Cycloid_R27_Rr3_N12_E1.3 v13 (Autodesk Fusion 360 design; units mm, degrees)
Autodesk Fusion 360 part; units mm, degrees
sketch "Cycloid_R27_Rr3_N12_E1.3" plane through (0, 0, 0) normal (0, 0, 1) x (1, 0, 0)
  spline S0 degree 3 poles (22.7, 0) (22.7, 0.6125) (22.8641, 1.1792) (23.0258, 1.5653) (23.2959, 2.21) (23.5195, 2.5021) (23.6979, 2.8113) (23.9582, 3.2623) (24.184, 3.7168) (24.3374, 4.3219) (24.5549, 5.1798) (24.5562, 6.3107) (24.2085, 7.3389) (23.915, 8.2071) (23.3942, 8.9658) (22.849, 9.4857) (22.4062, 9.9079) (21.976, 10.1744) (21.5331, 10.4069) (21.2661, 10.5471) (20.9901, 10.6664) (20.5771, 10.9051) (20.2716, 11.0818) (19.8561, 11.3456) (19.4485, 11.8071) (19.0699, 12.2358) (18.7698, 12.8235) (18.6313, 13.3021) (18.4366, 13.9744) (18.4464, 14.4072) (18.4331, 14.7458) (18.4124, 15.2731) (18.4019, 15.6633) (18.3082, 16.1442) (18.1696, 16.8555) (17.8268, 17.7143) (17.2032, 18.47) (16.54, 19.2736) (15.5782, 19.8983) (14.6774, 20.1844) (14.0278, 20.3907) (13.4343, 20.4394) (12.9166, 20.4231) (12.5338, 20.411) (12.2077, 20.3607) (11.6984, 20.3178) (11.348, 20.2882) (10.8614, 20.2427) (10.1869, 20.3943) (9.6219, 20.5214) (8.984, 20.8456) (8.564, 21.1934) (8.0345, 21.632) (7.7911, 22.0076) (7.5955, 22.2842) (7.2871, 22.7202) (7.0844, 23.0287) (6.7768, 23.3686) (6.3145, 23.8797) (5.6298, 24.415) (4.747, 24.748) (3.7861, 25.1104) (2.6334, 25.1828) (1.6851, 24.9763) (1.0227, 24.8321) (0.4702, 24.5758) (0.0307, 24.2999) (-0.3331, 24.0715) (-0.6042, 23.843) (-0.9968, 23.5316) (-1.2336, 23.3438) (-1.5241, 23.0997) (-2.0364, 22.845) (-2.4624, 22.6331) (-3.0792, 22.4489) (-3.6623, 22.4317) (-4.2859, 22.4133) (-4.7902, 22.5464) (-5.1412, 22.6614) (-5.7453, 22.8593) (-6.0464, 23.0205) (-6.4003, 23.1512) (-6.9273, 23.3459) (-7.5288, 23.5011) (-8.2685, 23.5031) (-9.1925, 23.5056) (-10.2849, 23.2163) (-11.164, 22.6594) (-11.975, 22.1456) (-12.5739, 21.4439) (-12.9316, 20.8087) (-13.1579, 20.4068) (-13.2952, 20.0445) (-13.4326, 19.6384) (-13.5351, 19.3355) (-13.6176, 18.9984) (-13.88, 18.4589) (-14.0614, 18.0859) (-14.3743, 17.5893) (-14.8368, 17.1805) (-15.3004, 16.7706) (-15.8457, 16.5145) (-16.2496, 16.3807) (-16.9256, 16.1568) (-17.2959, 16.1359) (-17.6504, 16.0674) (-18.1624, 15.9683) (-18.6562, 15.8398) (-19.2159, 15.5567) (-19.9761, 15.1721) (-20.7954, 14.4746) (-21.3419, 13.5856) (-21.8985, 12.6803) (-22.1404, 11.6323) (-22.1375, 10.7953) (-22.1357, 10.2824) (-22.0608, 9.8568) (-21.9594, 9.4298) (-21.8808, 9.099) (-21.7667, 8.7789) (-21.6764, 8.1745) (-21.6194, 7.793) (-21.5831, 7.2498) (-21.7151, 6.6502) (-21.8449, 6.0605) (-22.143, 5.5032) (-22.4147, 5.1385) (-22.8549, 4.5478) (-23.1744, 4.3137) (-23.4331, 4.0707) (-23.8211, 3.7064) (-24.1569, 3.3625) (-24.4808, 2.8538) (-24.9221, 2.1607) (-25.272, 1.1745) (-25.2982, 0.1386) (-25.3223, -0.8106) (-25.0739, -1.7578) (-24.7014, -2.4719) (-24.3965, -3.0566) (-24.0398, -3.477) (-23.6716, -3.8416) (-23.4461, -4.065) (-23.2125, -4.2595) (-22.876, -4.6039) (-22.6373, -4.8482) (-22.3173, -5.1939) (-22.0405, -5.74) (-21.7861, -6.2422) (-21.6353, -6.8982) (-21.625, -7.4159) (-21.6112, -8.1077) (-21.7373, -8.5368) (-21.8186, -8.8665) (-21.9475, -9.3885) (-22.0486, -9.7489) (-22.1025, -10.2133) (-22.1829, -10.9066) (-22.1299, -11.7884) (-21.7892, -12.6793) (-21.4199, -13.6452) (-20.7045, -14.5555) (-19.9227, -15.1243) (-19.3974, -15.5065) (-18.8642, -15.7434) (-18.3853, -15.8897) (-17.9769, -16.0144) (-17.6277, -16.07) (-17.1406, -16.1615) (-16.8439, -16.2172) (-16.4707, -16.276) (-15.9426, -16.4947) (-15.5053, -16.6757) (-14.9625, -17.0173) (-14.5654, -17.4455) (-14.1421, -17.9021) (-13.9093, -18.3711) (-13.765, -18.7126) (-13.5164, -19.301) (-13.4413, -19.6348) (-13.3093, -19.987) (-13.1131, -20.5104) (-12.8409, -21.0621) (-12.3647, -21.6203) (-11.7686, -22.3192) (-10.8433, -22.9587) (-9.8503, -23.2649) (-8.9138, -23.5536) (-7.9704, -23.5471) (-7.2443, -23.3971) (-6.7961, -23.3044) (-6.4349, -23.1714) (-6.0396, -23.0098) (-5.7254, -22.8814) (-5.397, -22.7049) (-4.742, -22.5476) (-4.3177, -22.4458) (-3.7077, -22.3819) (-3.1052, -22.4891) (-2.4937, -22.5979) (-1.9804, -22.8541) (-1.6382, -23.069) (-1.0631, -23.4303) (-0.813, -23.6841) (-0.5276, -23.9055) (-0.0967, -24.2396) (0.3681, -24.5462) (1.0085, -24.7802) (1.8665, -25.0938) (3.0127, -25.2008) (4.0658, -24.9549) (4.945, -24.7496) (5.7243, -24.3197) (6.2774, -23.8522) (6.7357, -23.4649) (7.0339, -23.0841) (7.3327, -22.66) (7.5073, -22.4123) (7.6728, -22.1364) (8.0197, -21.732) (8.2737, -21.436) (8.6677, -21.048) (9.2148, -20.7552) (9.7556, -20.4658) (10.3782, -20.3321) (10.8314, -20.3024) (11.5372, -20.2561) (11.9151, -20.3387) (12.2602, -20.3744) (12.7705, -20.4273) (13.2294, -20.4562) (13.7969, -20.3811) (14.601, -20.2747) (15.574, -19.9156) (16.3855, -19.2718) (17.1618, -18.6559) (17.7486, -17.8083) (18.0529, -17.027) (18.2904, -16.4172) (18.3721, -15.8769) (18.4057, -15.3617) (18.4274, -15.0299) (18.417, -14.7129) (18.468, -14.1849) (18.5019, -13.8331) (18.5698, -13.3444) (18.8214, -12.7816) (19.0638, -12.2391) (19.4972, -11.7071) (19.886, -11.3825) (20.4355, -10.9236) (20.8302, -10.7624) (21.1363, -10.6086) (21.5943, -10.3785) (21.9506, -10.1986) (22.3517, -9.903) (22.9505, -9.4617) (23.5934, -8.7583) (24.0064, -7.8502) (24.438, -6.9014) (24.5746, -5.7752) (24.443, -4.8563) (24.3415, -4.1467) (24.1137, -3.5815) (23.8589, -3.1009) (23.7019, -2.8048) (23.5323, -2.548) (23.3033, -2.1326) (23.1455, -1.8464) (22.9357, -1.4585) (22.8, -0.8709) (22.7389, -0.6059) (22.7, -0.3041) (22.7, 0) knots 0 0 0 0 0.03430611 0.03430611 0.03430611 0.09160089 0.09160089 0.09160089 0.17516843 0.17516843 0.17516843 0.29364805 0.29364805 0.29364805 0.39367837 0.39367837 0.39367837 0.47491142 0.47491142 0.47491142 0.5238857 0.5238857 0.5238857 0.5601117 0.5601117 0.5601117 0.59375346 0.59375346 0.59375346 0.64102096 0.64102096 0.64102096 0.71462274 0.71462274 0.71462274 0.82350645 0.82350645 0.82350645 0.93929104 0.93929104 0.93929104 1.02278938 1.02278938 1.02278938 1.08452204 1.08452204 1.08452204 1.12698868 1.12698868 1.12698868 1.16256928 1.16256928 1.16256928 1.2074329 1.2074329 1.2074329 1.27813427 1.27813427 1.27813427 1.38442402 1.38442402 1.38442402 1.50011681 1.50011681 1.50011681 1.58093887 1.58093887 1.58093887 1.64783508 1.64783508 1.64783508 1.68819847 1.68819847 1.68819847 1.72176401 1.72176401 1.72176401 1.75766421 1.75766421 1.75766421 1.81944996 1.81944996 1.81944996 1.91144577 1.91144577 1.91144577 2.02636364 2.02636364 2.02636364 2.13238209 2.13238209 2.13238209 2.19946819 2.19946819 2.19946819 2.24950351 2.24950351 2.24950351 2.28408659 2.28408659 2.28408659 2.31875688 2.31875688 2.31875688 2.37677319 2.37677319 2.37677319 2.46056379 2.46056379 2.46056379 2.57436902 2.57436902 2.57436902 2.69026953 2.69026953 2.69026953 2.7613022 2.7613022 2.7613022 2.81633163 2.81633163 2.81633163 2.85106272 2.85106272 2.85106272 2.88522235 2.88522235 2.88522235 2.94055461 2.94055461 2.94055461 3.02352207 3.02352207 3.02352207 3.13655488 3.13655488 3.13655488 3.24012125 3.24012125 3.24012125 3.32490764 3.32490764 3.32490764 3.37684352 3.37684352 3.37684352 3.413689 3.413689 3.413689 3.44756834 3.44756834 3.44756834 3.49284999 3.49284999 3.49284999 3.56456328 3.56456328 3.56456328 3.67163442 3.67163442 3.67163442 3.78772273 3.78772273 3.78772273 3.86570593 3.86570593 3.86570593 3.93220732 3.93220732 3.93220732 3.97271018 3.97271018 3.97271018 4.00624962 4.00624962 4.00624962 4.04200453 4.04200453 4.04200453 4.10360991 4.10360991 4.10360991 4.19515686 4.19515686 4.19515686 4.30976018 4.30976018 4.30976018 4.41784404 4.41784404 4.41784404 4.48458241 4.48458241 4.48458241 4.53760721 4.53760721 4.53760721 4.57196123 4.57196123 4.57196123 4.60683368 4.60683368 4.60683368 4.66544576 4.66544576 4.66544576 4.75391117 4.75391117 4.75391117 4.87242781 4.87242781 4.87242781 4.9713785 4.9713785 4.9713785 5.05336643 5.05336643 5.05336643 5.10124548 5.10124548 5.10124548 5.1362929 5.1362929 5.1362929 5.17093432 5.17093432 5.17093432 5.22489121 5.22489121 5.22489121 5.30468399 5.30468399 5.30468399 5.41776894 5.41776894 5.41776894 5.52594598 5.52594598 5.52594598 5.61037845 5.61037845 5.61037845 5.66476024 5.66476024 5.66476024 5.70099726 5.70099726 5.70099726 5.7359224 5.7359224 5.7359224 5.78528307 5.78528307 5.78528307 5.85915785 5.85915785 5.85915785 5.96942398 5.96942398 5.96942398 6.08463245 6.08463245 6.08463245 6.17359078 6.17359078 6.17359078 6.22838805 6.22838805 6.22838805 6.26615392 6.26615392 6.26615392 6.28318531 6.28318531 6.28318531 6.28318531
  circle A0 centre (0, 0) radius 9.1
  circle A1 centre (0, 0) radius 16 construction
  line L0 (0, 0) -> (0, 22.3554) construction
  circle A2 centre (0, 16) radius 4.3
  circle A3 centre (-15.2169, 4.9443) radius 4.3
  circle A4 centre (-9.4046, -12.9443) radius 4.3
  circle A5 centre (9.4046, -12.9443) radius 4.3
  circle A6 centre (15.2169, 4.9443) radius 4.3
  circle A7 centre (0, 0) radius 8
  dimension "d13" = 18.2
  dimension "d14" = 8.6
  dimension "d16" = 360
  dimension "d17" = 16
  dimension "d28" = 32
  constraint coincident A0.centre A1.centre
  constraint vertical L0
  constraint coincident A1 A2.centre
  constraint coincident L0 A2.centre
  constraint concentric A0 A7
  measures "d13" diameter of A0
  measures "d14" diameter of A2
  measures "d17" diameter of A7
  measures "d28" diameter of A1
extrude "Extrude3" add sketch "Cycloid_R27_Rr3_N12_E1.3" along normal blind 8 contours S0 makes body 1
extrude "Extrude4" add sketch "Cycloid_R27_Rr3_N12_E1.3" along normal blind 1.8 contours A0 bodies 1
sketch "Sketch4" plane through (0, 0, 8) normal (0, 0, 1) x (-1, 0, 0)
  circle A0 centre (0, 0) radius 9.1
  circle A1 centre (9.4046, 12.9443) radius 4.3
  circle A2 centre (15.2169, -4.9443) radius 4.3
  circle A3 centre (0, -16) radius 4.3
  circle A4 centre (-9.4046, 12.9443) radius 4.3
  circle A5 centre (-15.2169, -4.9443) radius 4.3
  spline S0 degree 3 poles (-22.7, 0) (-22.7, -0.6125) (-22.8641, -1.1792) (-23.0258, -1.5653) (-23.2959, -2.21) (-23.5195, -2.5021) (-23.6979, -2.8113) (-23.9582, -3.2623) (-24.184, -3.7168) (-24.3374, -4.3219) (-24.5549, -5.1798) (-24.5562, -6.3107) (-24.2085, -7.3389) (-23.915, -8.2071) (-23.3942, -8.9658) (-22.849, -9.4857) (-22.4062, -9.9079) (-21.976, -10.1744) (-21.5331, -10.4069) (-21.2661, -10.5471) (-20.9901, -10.6664) (-20.5771, -10.9051) (-20.2716, -11.0818) (-19.8561, -11.3456) (-19.4485, -11.8071) (-19.0699, -12.2358) (-18.7698, -12.8235) (-18.6313, -13.3021) (-18.4366, -13.9744) (-18.4464, -14.4072) (-18.4331, -14.7458) (-18.4124, -15.2731) (-18.4019, -15.6633) (-18.3082, -16.1442) (-18.1696, -16.8555) (-17.8268, -17.7143) (-17.2032, -18.47) (-16.54, -19.2736) (-15.5782, -19.8983) (-14.6774, -20.1844) (-14.0278, -20.3907) (-13.4343, -20.4394) (-12.9166, -20.4231) (-12.5338, -20.411) (-12.2077, -20.3607) (-11.6984, -20.3178) (-11.348, -20.2882) (-10.8614, -20.2427) (-10.1869, -20.3943) (-9.6219, -20.5214) (-8.984, -20.8456) (-8.564, -21.1934) (-8.0345, -21.632) (-7.7911, -22.0076) (-7.5955, -22.2842) (-7.2871, -22.7202) (-7.0844, -23.0287) (-6.7768, -23.3686) (-6.3145, -23.8797) (-5.6298, -24.415) (-4.747, -24.748) (-3.7861, -25.1104) (-2.6334, -25.1828) (-1.6851, -24.9763) (-1.0227, -24.8321) (-0.4702, -24.5758) (-0.0307, -24.2999) (0.3331, -24.0715) (0.6042, -23.843) (0.9968, -23.5316) (1.2336, -23.3438) (1.5241, -23.0997) (2.0364, -22.845) (2.4624, -22.6331) (3.0792, -22.4489) (3.6623, -22.4317) (4.2859, -22.4133) (4.7902, -22.5464) (5.1412, -22.6614) (5.7453, -22.8593) (6.0464, -23.0205) (6.4003, -23.1512) (6.9273, -23.3459) (7.5288, -23.5011) (8.2685, -23.5031) (9.1925, -23.5056) (10.2849, -23.2163) (11.164, -22.6594) (11.975, -22.1456) (12.5739, -21.4439) (12.9316, -20.8087) (13.1579, -20.4068) (13.2952, -20.0445) (13.4326, -19.6384) (13.5351, -19.3355) (13.6176, -18.9984) (13.88, -18.4589) (14.0614, -18.0859) (14.3743, -17.5893) (14.8368, -17.1805) (15.3004, -16.7706) (15.8457, -16.5145) (16.2496, -16.3807) (16.9256, -16.1568) (17.2959, -16.1359) (17.6504, -16.0674) (18.1624, -15.9683) (18.6562, -15.8398) (19.2159, -15.5567) (19.9761, -15.1721) (20.7954, -14.4746) (21.3419, -13.5856) (21.8985, -12.6803) (22.1404, -11.6323) (22.1375, -10.7953) (22.1357, -10.2824) (22.0608, -9.8568) (21.9594, -9.4298) (21.8808, -9.099) (21.7667, -8.7789) (21.6764, -8.1745) (21.6194, -7.793) (21.5831, -7.2498) (21.7151, -6.6502) (21.8449, -6.0605) (22.143, -5.5032) (22.4147, -5.1385) (22.8549, -4.5478) (23.1744, -4.3137) (23.4331, -4.0707) (23.8211, -3.7064) (24.1569, -3.3625) (24.4808, -2.8538) (24.9221, -2.1607) (25.272, -1.1745) (25.2982, -0.1386) (25.3223, 0.8106) (25.0739, 1.7578) (24.7014, 2.4719) (24.3965, 3.0566) (24.0398, 3.477) (23.6716, 3.8416) (23.4461, 4.065) (23.2125, 4.2595) (22.876, 4.6039) (22.6373, 4.8482) (22.3173, 5.1939) (22.0405, 5.74) (21.7861, 6.2422) (21.6353, 6.8982) (21.625, 7.4159) (21.6112, 8.1077) (21.7373, 8.5368) (21.8186, 8.8665) (21.9475, 9.3885) (22.0486, 9.7489) (22.1025, 10.2133) (22.1829, 10.9066) (22.1299, 11.7884) (21.7892, 12.6793) (21.4199, 13.6452) (20.7045, 14.5555) (19.9227, 15.1243) (19.3974, 15.5065) (18.8642, 15.7434) (18.3853, 15.8897) (17.9769, 16.0144) (17.6277, 16.07) (17.1406, 16.1615) (16.8439, 16.2172) (16.4707, 16.276) (15.9426, 16.4947) (15.5053, 16.6757) (14.9625, 17.0173) (14.5654, 17.4455) (14.1421, 17.9021) (13.9093, 18.3711) (13.765, 18.7126) (13.5164, 19.301) (13.4413, 19.6348) (13.3093, 19.987) (13.1131, 20.5104) (12.8409, 21.0621) (12.3647, 21.6203) (11.7686, 22.3192) (10.8433, 22.9587) (9.8503, 23.2649) (8.9138, 23.5536) (7.9704, 23.5471) (7.2443, 23.3971) (6.7961, 23.3044) (6.4349, 23.1714) (6.0396, 23.0098) (5.7254, 22.8814) (5.397, 22.7049) (4.742, 22.5476) (4.3177, 22.4458) (3.7077, 22.3819) (3.1052, 22.4891) (2.4937, 22.5979) (1.9804, 22.8541) (1.6382, 23.069) (1.0631, 23.4303) (0.813, 23.6841) (0.5276, 23.9055) (0.0967, 24.2396) (-0.3681, 24.5462) (-1.0085, 24.7802) (-1.8665, 25.0938) (-3.0127, 25.2008) (-4.0658, 24.9549) (-4.945, 24.7496) (-5.7243, 24.3197) (-6.2774, 23.8522) (-6.7357, 23.4649) (-7.0339, 23.0841) (-7.3327, 22.66) (-7.5073, 22.4123) (-7.6728, 22.1364) (-8.0197, 21.732) (-8.2737, 21.436) (-8.6677, 21.048) (-9.2148, 20.7552) (-9.7556, 20.4658) (-10.3782, 20.3321) (-10.8314, 20.3024) (-11.5372, 20.2561) (-11.9151, 20.3387) (-12.2602, 20.3744) (-12.7705, 20.4273) (-13.2294, 20.4562) (-13.7969, 20.3811) (-14.601, 20.2747) (-15.574, 19.9156) (-16.3855, 19.2718) (-17.1618, 18.6559) (-17.7486, 17.8083) (-18.0529, 17.027) (-18.2904, 16.4172) (-18.3721, 15.8769) (-18.4057, 15.3617) (-18.4274, 15.0299) (-18.417, 14.7129) (-18.468, 14.1849) (-18.5019, 13.8331) (-18.5698, 13.3444) (-18.8214, 12.7816) (-19.0638, 12.2391) (-19.4972, 11.7071) (-19.886, 11.3825) (-20.4355, 10.9236) (-20.8302, 10.7624) (-21.1363, 10.6086) (-21.5943, 10.3785) (-21.9506, 10.1986) (-22.3517, 9.903) (-22.9505, 9.4617) (-23.5934, 8.7583) (-24.0064, 7.8502) (-24.438, 6.9014) (-24.5746, 5.7752) (-24.443, 4.8563) (-24.3415, 4.1467) (-24.1137, 3.5815) (-23.8589, 3.1009) (-23.7019, 2.8048) (-23.5323, 2.548) (-23.3033, 2.1326) (-23.1455, 1.8464) (-22.9357, 1.4585) (-22.8, 0.8709) (-22.7389, 0.6059) (-22.7, 0.3041) (-22.7, 0) knots 0 0 0 0 0.03430611 0.03430611 0.03430611 0.09160089 0.09160089 0.09160089 0.17516843 0.17516843 0.17516843 0.29364805 0.29364805 0.29364805 0.39367837 0.39367837 0.39367837 0.47491142 0.47491142 0.47491142 0.5238857 0.5238857 0.5238857 0.5601117 0.5601117 0.5601117 0.59375346 0.59375346 0.59375346 0.64102096 0.64102096 0.64102096 0.71462274 0.71462274 0.71462274 0.82350645 0.82350645 0.82350645 0.93929104 0.93929104 0.93929104 1.02278938 1.02278938 1.02278938 1.08452204 1.08452204 1.08452204 1.12698868 1.12698868 1.12698868 1.16256928 1.16256928 1.16256928 1.2074329 1.2074329 1.2074329 1.27813427 1.27813427 1.27813427 1.38442402 1.38442402 1.38442402 1.50011681 1.50011681 1.50011681 1.58093887 1.58093887 1.58093887 1.64783508 1.64783508 1.64783508 1.68819847 1.68819847 1.68819847 1.72176401 1.72176401 1.72176401 1.75766421 1.75766421 1.75766421 1.81944996 1.81944996 1.81944996 1.91144577 1.91144577 1.91144577 2.02636364 2.02636364 2.02636364 2.13238209 2.13238209 2.13238209 2.19946819 2.19946819 2.19946819 2.24950351 2.24950351 2.24950351 2.28408659 2.28408659 2.28408659 2.31875688 2.31875688 2.31875688 2.37677319 2.37677319 2.37677319 2.46056379 2.46056379 2.46056379 2.57436902 2.57436902 2.57436902 2.69026953 2.69026953 2.69026953 2.7613022 2.7613022 2.7613022 2.81633163 2.81633163 2.81633163 2.85106272 2.85106272 2.85106272 2.88522235 2.88522235 2.88522235 2.94055461 2.94055461 2.94055461 3.02352207 3.02352207 3.02352207 3.13655488 3.13655488 3.13655488 3.24012125 3.24012125 3.24012125 3.32490764 3.32490764 3.32490764 3.37684352 3.37684352 3.37684352 3.413689 3.413689 3.413689 3.44756834 3.44756834 3.44756834 3.49284999 3.49284999 3.49284999 3.56456328 3.56456328 3.56456328 3.67163442 3.67163442 3.67163442 3.78772273 3.78772273 3.78772273 3.86570593 3.86570593 3.86570593 3.93220732 3.93220732 3.93220732 3.97271018 3.97271018 3.97271018 4.00624962 4.00624962 4.00624962 4.04200453 4.04200453 4.04200453 4.10360991 4.10360991 4.10360991 4.19515686 4.19515686 4.19515686 4.30976018 4.30976018 4.30976018 4.41784404 4.41784404 4.41784404 4.48458241 4.48458241 4.48458241 4.53760721 4.53760721 4.53760721 4.57196123 4.57196123 4.57196123 4.60683368 4.60683368 4.60683368 4.66544576 4.66544576 4.66544576 4.75391117 4.75391117 4.75391117 4.87242781 4.87242781 4.87242781 4.9713785 4.9713785 4.9713785 5.05336643 5.05336643 5.05336643 5.10124548 5.10124548 5.10124548 5.1362929 5.1362929 5.1362929 5.17093432 5.17093432 5.17093432 5.22489121 5.22489121 5.22489121 5.30468399 5.30468399 5.30468399 5.41776894 5.41776894 5.41776894 5.52594598 5.52594598 5.52594598 5.61037845 5.61037845 5.61037845 5.66476024 5.66476024 5.66476024 5.70099726 5.70099726 5.70099726 5.7359224 5.7359224 5.7359224 5.78528307 5.78528307 5.78528307 5.85915785 5.85915785 5.85915785 5.96942398 5.96942398 5.96942398 6.08463245 6.08463245 6.08463245 6.17359078 6.17359078 6.17359078 6.22838805 6.22838805 6.22838805 6.26615392 6.26615392 6.26615392 6.28318531 6.28318531 6.28318531 6.28318531
  circle A6 centre (0, 0) radius 10.5
  dimension "d22" = 21
  constraint concentric A0 A6
  measures "d22" diameter of A6
extrude "Extrude5" cut sketch "Sketch4" against normal blind 2 contours A6 bodies 1
sketch "Sketch1" plane through (0, 0, 6) normal (0, 0, 1) x (-1, 0, 0) in component "Cover"
  circle A0 centre (0, 0) radius 9.1
  circle A1 centre (0, 0) radius 10.5
  circle A2 centre (0, 0) radius 8
  dimension "d25" = 16
  constraint concentric A0 A2
  measures "d25" diameter of A2
extrude "Extrude1" add sketch "Sketch1" along normal blind 2 separate body contours A0 | A1 makes body 2 in component "Cover"
component "Cover" placed x (1, 0, 0) y (0, 1, 0) z (0, 0, 1) at (0, 0, 0)
equation "d14 = 6 mm + ( 2 * 1.3 ) * 1 mm"
